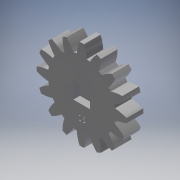
# Autodesk Inventor part: 16_teeth
Saved by Autodesk Inventor 2019 (Build 230136000, 136)
## iProperties
Created: 2020-02-24
Part Number: 16_teeth
Material: Steel
Document SubType Name: Modeling
Designer: Jeff
Categories: <?xml version="1.0" encoding="UTF-16"?> <MemberInstance><Categories><FamilyTemplate><FamilyTemplateParameter ValueType="xs:double" Id="1" ObjectReferenceKey="da_z" ObjectType="kUserParameterObject"/><FamilyTemplateParameter ValueType="xs:double" Id="2" ObjectReferenceKey="da_b" ObjectType="kUserParameterObject"/><FamilyTemplateParameter ValueType="xs:double" Id="3" ObjectReferenceKey="da_beta" ObjectType="kUserParameterObject"/><FamilyTemplateParameter ValueType="xs:double" Id="4" ObjectReferenceKey="da_da" ObjectType="kUserParameterObject"/><FamilyTemplateParameter ValueType="xs:double" Id="5" ObjectReferenceKey="da_aw" ObjectType="kUserParameterObject"/><FamilyTemplateParameter ValueType="xs:string" Id="6" ObjectReferenceKey="EAIAABAAAACIAQAAAAAAAIAAAAAAAAAA" ObjectType="83910656" SubObjectId="SurfaceGeometry"/></FamilyTemplate><ParamToTemplateMap><ParamToTemplate CategoryParameter="//CategoryParameter[@InternalName='046C89C9-8512-4d59-83FE-43B91F4F132A']" TemplateParameter="1"/><ParamToTemplate CategoryParameter="//CategoryParameter[@InternalName='2552DF32-E462-4b46-AEBF-C6C7768E72AC']" TemplateParameter="2"/><ParamToTemplate CategoryParameter="//CategoryParameter[@InternalName='C9EE641D-15FC-4fae-A226-E94C4372FDD7']" TemplateParameter="3"/><ParamToTemplate><ParamToTemplate CategoryParameter="//CategoryParameter[@InternalName='00B6519A-459B-49c7-AD84-2E56D39A5744']" ConstantValue="0.000000"/></ParamToTemplate><ParamToTemplate><ParamToTemplate CategoryParameter="//CategoryParameter[@InternalName='04B31F0E-C7A6-4894-AA32-9629BEFACF47']" ConstantValue="1.000000"/></ParamToTemplate><ParamToTemplate><ParamToTemplate CategoryParameter="//CategoryParameter[@InternalName='43CBEC2E-7847-49e7-A936-2F7889FCB2D9']" ConstantValue="0.250000"/></ParamToTemplate><ParamToTemplate><ParamToTemplate CategoryParameter="//CategoryParameter[@InternalName='B1EFC894-105D-4ebd-86BF-FA20ED196853']" ConstantValue="0.350000"/></ParamToTemplate><ParamToTemplate><ParamToTemplate CategoryParameter="//CategoryParameter[@InternalName='51175063-3D10-4879-93E8-6246FE8B403D']" ConstantValue="2060000000.000000"/></ParamToTemplate><ParamToTemplate><ParamToTemplate CategoryParameter="//CategoryParameter[@InternalName='A3A52E27-4454-46a9-B0BD-C932399B70AF']" ConstantValue="0.300000"/></ParamToTemplate><ParamToTemplate><ParamToTemplate CategoryParameter="//CategoryParameter[@InternalName='91B76062-C214-41d9-B1B9-14D2AB99603D']" ConstantValue="0.300000"/></ParamToTemplate><ParamToTemplate><ParamToTemplate CategoryParameter="//CategoryParameter[@InternalName='374E806E-8B8A-4dda-A9AA-1039D6500AD2']" ConstantValue="3.333333"/></ParamToTemplate><ParamToTemplate><ParamToTemplate CategoryParameter="//CategoryParameter[@InternalName='2D373A89-B862-43d6-8D0B-0CBF12AB9F6C']" ConstantValue="0.349066"/></ParamToTemplate><ParamToTemplate CategoryParameter="//CategoryParameter[@InternalName='37777632-D6A2-4fac-9D53-DB8ACD95C989']" TemplateParameter="4"/><ParamToTemplate CategoryParameter="//CategoryParameter[@InternalName='FD1017F1-B727-4f7e-9707-0F86F1FF9423']" TemplateParameter="5"/><ParamToTemplate><ParamToTemplate CategoryParameter="//CategoryParameter[@InternalName='9E1B4470-B2D3-4ff1-B813-535BB4CDF51A']" ConstantValue="3520000.000000"/></ParamToTemplate><ParamToTemplate><ParamToTemplate CategoryParameter="//CategoryParameter[@InternalName='F8452263-BFF6-458c-9FB1-07C4B99E95CD']" ConstantValue="11400000.000000"/></ParamToTemplate><ParamToTemplate><ParamToTemplate CategoryParameter="//CategoryParameter[@InternalName='3E3BB259-FD49-497f-8171-6EBC954A3479']" ConstantValue="2.000000"/></ParamToTemplate><ParamToTemplate CategoryParameter="//CategoryParameter[@InternalName='27C3BAF2-7550-4e4b-AE2C-0DB134B7D9B7']" TemplateParameter="6"/></ParamToTemplateMap><Category DisplayName="Gear" InternalName="DC85795E-93AB-48d5-8EEE-5A27447B64BD" Mnemonic="Gear"><CategoryParameter DisplayName="z" InternalName="046C89C9-8512-4d59-83FE-43B91F4F132A" Mnemonic="z"/><CategoryParameter DisplayName="b" InternalName="2552DF32-E462-4b46-AEBF-C6C7768E72AC" Mnemonic="b"/><CategoryParameter DisplayName="||b|" InternalName="C9EE641D-15FC-4fae-A226-E94C4372FDD7" Mnemonic="beta"/><CategoryParameter DisplayName="x" InternalName="00B6519A-459B-49c7-AD84-2E56D39A5744" Mnemonic="x"/><CategoryParameter DisplayName="a*" InternalName="04B31F0E-C7A6-4894-AA32-9629BEFACF47" Mnemonic="a"/><CategoryParameter DisplayName="c*" InternalName="43CBEC2E-7847-49e7-A936-2F7889FCB2D9" Mnemonic="c"/><CategoryParameter DisplayName="r|.f|*" InternalName="B1EFC894-105D-4ebd-86BF-FA20ED196853" Mnemonic="rf"/><CategoryParameter DisplayName="E" InternalName="51175063-3D10-4879-93E8-6246FE8B403D" Mnemonic="E"/><CategoryParameter DisplayName="||m|" InternalName="A3A52E27-4454-46a9-B0BD-C932399B70AF" Mnemonic="mi"/><Category DisplayName="SpurGear" InternalName="26C5A22E-A91E-4dfd-A3B3-23CCAFAE1764" Mnemonic="SpurGear"><CategoryParameter DisplayName="m" InternalName="91B76062-C214-41d9-B1B9-14D2AB99603D" Mnemonic="m"/><CategoryParameter DisplayName="P" InternalName="374E806E-8B8A-4dda-A9AA-1039D6500AD2" Mnemonic="PP"/><CategoryParameter DisplayName="||a|" InternalName="2D373A89-B862-43d6-8D0B-0CBF12AB9F6C" Mnemonic="alpha"/><CategoryParameter DisplayName="d|.a|" InternalName="37777632-D6A2-4fac-9D53-DB8ACD95C989" Mnemonic="da"/><CategoryParameter DisplayName="a|.w|" InternalName="FD1017F1-B727-4f7e-9707-0F86F1FF9423" Mnemonic="aw"/><CategoryParameter DisplayName="||s||.Flim|" InternalName="9E1B4470-B2D3-4ff1-B813-535BB4CDF51A" Mnemonic="sFlim"/><CategoryParameter DisplayName="||s||.Hlim|" InternalName="F8452263-BFF6-458c-9FB1-07C4B99E95CD" Mnemonic="sHlim"/><CategoryParameter DisplayName="type" InternalName="3E3BB259-FD49-497f-8171-6EBC954A3479" Mnemonic="type"/><CategoryParameter DisplayName="PitchDiameter" InternalName="27C3BAF2-7550-4e4b-AE2C-0DB134B7D9B7" Mnemonic="IDS_PITCHDIAM"/></Category></Category></Categories></MemberInstance>
Density: 1 g/cm^3
Appearance: Steel
CustomPartVersion: 1
Author: Jeff
Autodesk Inventor part; units mm, degrees
sketch "Sketch1" plane through (0, 0, 0) normal (0, 0, 1) x (1, 0, 0)
  circle A0 centre (0, 0) radius 27
  dimension "d0" = 54
  constraints: 1 centre point
  measures "d0" diameter of A0
extrude "Extrusion1" add sketch "Sketch1" along normal blind 10
ref_plane "Work Plane2" through (0, 0, 5) normal (0, 0, 1) x (1, 0, 0)
sketch "Sketch2" plane through (0, 0, 0) normal (0, 0, -1) x (-1, 0, 0)
  circle A0 centre (0, 0) radius 27 projected
  circle A1 centre (0, 0) radius 24
  dimension "d3" = 48
  constraints: 1 centre point, 1 coincident
  measures "d3" diameter of A1
surface extrude "Pitch Diameter" sketch "Sketch2" against normal through all shown no curves A1
ref_plane "Work Plane8" through (0, 0, 0) normal (0.9807853, 0.1950903, 0) x (0, 0, 1)
ref_plane "Work Plane9" through (0, 0, 0) normal (1, 0, 0) x (0, 1, 0)
spur gear teeth "Spur Gear" teeth 16 pitch diameter 48 tip diameter 54 root diameter 40.5 face width 10 start plane through (0, 0, 0) normal (0, 0, -1) x (-1, 0, 0)
sketch "Sketch3" plane through (0, 0, 10) normal (0, 0, 1) x (1, 0, 0)
  line L0 (-5, 5) -> (5, 5)
  line L1 (5, 5) -> (5, -5)
  line L2 (5, -5) -> (-5, -5)
  line L3 (-5, -5) -> (-5, 5)
  line L4 (-5, -17.5154) -> (-5, -7.5154) construction
  line L5 (-5, -7.5154) -> (5, -7.5154) construction
  line L6 (5, -7.5154) -> (5, -17.5154) construction
  line L7 (5, -17.5154) -> (-5, -17.5154) construction
  arc A0 (-2.9713, -20.0308) -> (-1.3248, -26.9675) centre (19.0094, -18.4773) ccw projected
  line L8 (-2.9713, -20.0308) -> (-2.9713, -5)
  line L9 (-0.3331, -14.0118) -> (-1.7966, -14.0118)
  line L10 (-1.7966, -14.0118) -> (-1.7966, -13.7054)
  line L11 (-1.7966, -13.7054) -> (-1.252, -13.7054)
  line L12 (-1.252, -13.7054) -> (-1.252, -11.6949)
  line L13 (-1.252, -11.6949) -> (-1.7966, -11.6949)
  line L14 (-1.7966, -11.6949) -> (-1.7966, -11.4202)
  spline S0 degree 2 poles (-1.7966, -11.4202) (-1.4878, -11.4202) (-1.1961, -11.2452) (-1.1767, -11.002) knots 0 0 0 1 2 2 2
  line L15 (-1.1767, -11.002) -> (-0.8655, -11.002)
  line L16 (-0.8655, -11.002) -> (-0.8655, -13.7054)
  line L17 (-0.8655, -13.7054) -> (-0.3331, -13.7054)
  line L18 (-0.3331, -13.7054) -> (-0.3331, -14.0118)
  spline S1 degree 2 poles (2.1151, -13.0393) (2.1151, -13.2703) (1.9619, -13.6617) (1.8331, -13.793) knots 0 0 0 1 2 2 2
  spline S2 degree 2 poles (1.8331, -13.793) (1.6994, -13.9315) (1.3639, -14.075) (1.1621, -14.075) knots 0 0 0 1 2 2 2
  spline S3 degree 2 poles (1.1621, -14.075) (0.9603, -14.075) (0.6272, -13.9388) (0.5008, -13.8027) knots 0 0 0 1 2 2 2
  spline S4 degree 2 poles (0.5008, -13.8027) (0.3452, -13.6398) (0.1702, -13.0928) (0.1702, -12.6941) knots 0 0 0 1 2 2 2
  spline S5 degree 2 poles (0.1702, -12.6941) (0.1702, -12.3027) (0.3306, -11.673) (0.4984, -11.4396) knots 0 0 0 1 2 2 2
  spline S6 degree 2 poles (0.4984, -11.4396) (0.6613, -11.2111) (1.1767, -10.9558) (1.5146, -10.9558) knots 0 0 0 1 2 2 2
  spline S7 degree 2 poles (1.5146, -10.9558) (1.6143, -10.9558) (1.7893, -10.9753) (1.8549, -10.9972) knots 0 0 0 1 2 2 2
  line L19 (1.8549, -10.9972) -> (1.8549, -11.3837)
  line L20 (1.8549, -11.3837) -> (1.8379, -11.3837)
  spline S8 degree 2 poles (1.8379, -11.3837) (1.782, -11.3546) (1.5778, -11.3035) (1.4611, -11.3035) knots 0 0 0 1 2 2 2
  spline S9 degree 2 poles (1.4611, -11.3035) (1.0867, -11.3035) (0.6272, -11.8092) (0.5835, -12.3051) knots 0 0 0 1 2 2 2
  spline S10 degree 2 poles (0.5835, -12.3051) (0.7269, -12.2054) (1.0284, -12.096) (1.2083, -12.096) knots 0 0 0 1 2 2 2
  spline S11 degree 2 poles (1.2083, -12.096) (1.3833, -12.096) (1.6459, -12.1665) (1.7893, -12.2735) knots 0 0 0 1 2 2 2
  spline S12 degree 2 poles (1.7893, -12.2735) (1.9546, -12.3975) (2.1151, -12.7816) (2.1151, -13.0393) knots 0 0 0 1 2 2 2
  spline S13 degree 2 poles (1.7066, -13.0563) (1.7066, -12.8716) (1.6094, -12.6212) (1.5024, -12.5336) knots 0 0 0 1 2 2 2
  spline S14 degree 2 poles (1.5024, -12.5336) (1.4222, -12.4704) (1.2229, -12.4291) (1.1183, -12.4291) knots 0 0 0 1 2 2 2
  spline S15 degree 2 poles (1.1183, -12.4291) (0.9773, -12.4291) (0.7123, -12.5142) (0.5835, -12.5944) knots 0 0 0 1 2 2 2
  spline S16 degree 2 poles (0.5835, -12.5944) (0.581, -12.6382) (0.5762, -12.7208) (0.5762, -12.7841) knots 0 0 0 1 2 2 2
  spline S17 degree 2 poles (0.5762, -12.7841) (0.5762, -13.0952) (0.6977, -13.4769) (0.7901, -13.5766) knots 0 0 0 1 2 2 2
  spline S18 degree 2 poles (0.7901, -13.5766) (0.8752, -13.6714) (1.06, -13.7468) (1.1645, -13.7468) knots 0 0 0 1 2 2 2
  spline S19 degree 2 poles (1.1645, -13.7468) (1.4076, -13.7468) (1.7066, -13.4016) (1.7066, -13.0563) knots 0 0 0 1 2 2 2
  point P0 (0, 0)
  point P1 (0, 5)
  point P2 (5, 0)
  point P3 (0, -7.5154)
  point P4 (-2.9713, -12.5154)
  point P5 (-5, -12.5154)
  dimension "d49" = 10
  dimension "d50" = 10
  dimension "d56" = 10
  dimension "d57" = 10
  constraints: 10 end point, 5 midpoint, 2 horizontal, 2 horizontal alignment, 2 parallel, 2 perpendicular, 1 point on line, 1 vertical alignment, 2 other
  measures "d49" distance of L1.end L2.end
  measures "d50" distance of L0.end L1.end
  measures "d56" distance between parallel lines of L6 L4
  measures "d57" distance between parallel lines of L5 L7
extrude "Extrusion2" cut sketch "Sketch3" against normal blind 4
sketch "Sketch4" plane through (0, 0, 0) normal (0, 0, -1) x (-1, 0, 0)
  circle A0 centre (0, 0) radius 7.5
  dimension "d53" = 15
  constraints: 1 centre point, 1 coincident
  measures "d53" diameter of A0
extrude "Extrusion3" cut sketch "Sketch4" against normal blind 4
equation "\"d0\" = da_da"
equation "\"d1\" = da_b"
equation "\"d3\" = da_dw"
equation "\"d16\" = da_aw"
equation "\"d43\" = da_aw"
equation "\"d46\" = da_aw"
equation "\"da_da\" = 54"
equation "\"da_b\" = 10"
equation "\"da_dw\" = 48"
equation "\"da_aw\" = 39"
body "Solid1"
body "Srf1"
